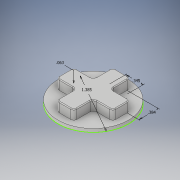
# Autodesk Inventor part: SnakeControllerDPad_v3
Saved by Autodesk Inventor 2019.1 (Build 231200000, 200)
## iProperties
Created: 2018-11-30
Part Number: SnakeControllerDPad_v3
Material: Generic
Document SubType Name: Modeling
Designer: Edward Hughes
Density: 1 g/cm^3
Appearance: Default
Author: Edward Hughes
Autodesk Inventor part; units mm, degrees
ref_plane "YZ Plane" through (0, 0, 0) normal (1, 0, 0) x (0, 1, 0)
ref_plane "XZ Plane" through (0, 0, 0) normal (0, 1, 0) x (-1, 0, 0)
ref_plane "XY Plane" through (0, 0, 0) normal (0, 0, 1) x (1, 0, 0)
sketch "Sketch1" plane through (0, 0, 0) normal (0, 1, 0) x (-1, 0, 0)
  circle A0 centre (0, 0) radius 17.5895
  line L0 (4.3815, 4.3815) -> (-4.3815, -4.3815) construction
  line L1 (-4.3815, 4.3815) -> (4.3815, -4.3815) construction
  line L2 (-4.3815, -5.969) -> (-4.3815, -12.5476)
  line L3 (-2.794, -14.1351) -> (2.794, -14.1351)
  line L4 (4.3815, -12.5476) -> (4.3815, -5.969)
  line L5 (-5.969, -4.3815) -> (-12.5476, -4.3815)
  line L6 (-14.1351, -2.794) -> (-14.1351, 2.794)
  line L7 (-12.5476, 4.3815) -> (-5.969, 4.3815)
  line L8 (4.3815, 5.969) -> (4.3815, 12.5476)
  line L9 (2.794, 14.1351) -> (-2.794, 14.1351)
  line L10 (-4.3815, 12.5476) -> (-4.3815, 5.969)
  line L11 (5.969, 4.3815) -> (12.5476, 4.3815)
  line L12 (14.1351, 2.794) -> (14.1351, -2.794)
  line L13 (12.5476, -4.3815) -> (5.969, -4.3815)
  arc A1 (12.5476, -4.3815) -> (14.1351, -2.794) centre (12.5476, -2.794) ccw
  arc A2 (5.969, -4.3815) -> (4.3815, -5.969) centre (5.969, -5.969) ccw
  arc A3 (2.794, -14.1351) -> (4.3815, -12.5476) centre (2.794, -12.5476) ccw
  arc A4 (-4.3815, -12.5476) -> (-2.794, -14.1351) centre (-2.794, -12.5476) ccw
  arc A5 (-4.3815, -5.969) -> (-5.969, -4.3815) centre (-5.969, -5.969) ccw
  arc A6 (-14.1351, -2.794) -> (-12.5476, -4.3815) centre (-12.5476, -2.794) ccw
  arc A7 (-12.5476, 4.3815) -> (-14.1351, 2.794) centre (-12.5476, 2.794) ccw
  arc A8 (-5.969, 4.3815) -> (-4.3815, 5.969) centre (-5.969, 5.969) ccw
  arc A9 (-2.794, 14.1351) -> (-4.3815, 12.5476) centre (-2.794, 12.5476) ccw
  arc A10 (4.3815, 12.5476) -> (2.794, 14.1351) centre (2.794, 12.5476) ccw
  arc A11 (4.3815, 5.969) -> (5.969, 4.3815) centre (5.969, 5.969) ccw
  arc A12 (14.1351, 2.794) -> (12.5476, 4.3815) centre (12.5476, 2.794) ccw
  point P0 (-4.3815, -14.1351)
  point P1 (-14.1351, 4.3815)
  point P2 (4.3815, 14.1351)
  point P3 (14.1351, -4.3815)
  dimension "d19" = 35.179
  dimension "d26" = 1.5875
  dimension "d27" = 9.7536
  dimension "d28" = 8.763
  constraints: 28 end point, 24 point on circle, 24 tangent, 13 centre point, 11 equal radius, 11 point on line, 4 parallel, 2 horizontal, 2 midpoint, 2 perpendicular
  measures "d19" diameter of A0
  measures "d26" radius of A1
  measures "d27" distance between parallel lines of L3 L5
  measures "d28" distance between parallel lines of L4 L2
extrude "Extrusion1" add sketch "Sketch1" along normal blind 6.35 contours A5 L5 A6 L6 A7 L7 A8 L10 A9 L9 A10 L8 A11 L11 A12 L12 A1 L13 A2 L4 A3 L3 A4 L2
extrude "Extrusion2" add sketch "Sketch1" along normal blind 1.5875
fillet "Fillet1" radius 0.3969 24 edges at (-4.8465, 6.35, 4.8465) (-4.3815, 6.35, 9.2583) (-3.9165, 6.35, 13.6701) (0, 6.35, 14.1351) (3.9165, 6.35, 13.6701) (4.3815, 6.35, 9.2583) (4.8465, 6.35, 4.8465) (9.2583, 6.35, 4.3815) (13.6701, 6.35, 3.9165) (14.1351, 6.35, 0) (13.6701, 6.35, -3.9165) (9.2583, 6.35, -4.3815) (4.8465, 6.35, -4.8465) (4.3815, 6.35, -9.2583) (3.9165, 6.35, -13.6701) (0, 6.35, -14.1351) (-3.9165, 6.35, -13.6701) (-4.3815, 6.35, -9.2583) (-4.8465, 6.35, -4.8465) (-9.2583, 6.35, -4.3815) (-13.6701, 6.35, -3.9165) (-14.1351, 6.35, 0) (-13.6701, 6.35, 3.9165) (-9.2583, 6.35, 4.3815)
body "Solid1"
